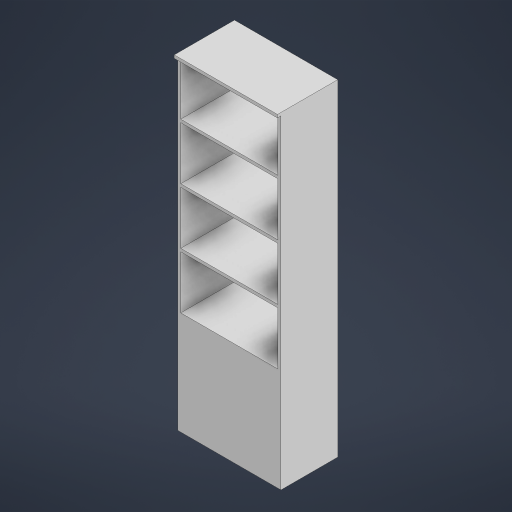
# Autodesk Inventor part: Libreria
Saved by Autodesk Inventor 2024.2 (Build 282272000, 272)
## iProperties
Created: 2025-08-11
Part Number: Libreria
Material: Generic
Document SubType Name: Modeling
Designer: Luca
Density: 1 g/cm^3
Appearance: Default
Author: Luca
Autodesk Inventor part; units mm, degrees
ref_plane "YZ Plane" through (0, 0, 0) normal (1, 0, 0) x (0, 1, 0)
ref_plane "XZ Plane" through (0, 0, 0) normal (0, 1, 0) x (-1, 0, 0)
ref_plane "XY Plane" through (0, 0, 0) normal (0, 0, 1) x (1, 0, 0)
sketch "Sketch1" plane through (0, 0, 0) normal (0, 0, 1) x (1, 0, 0)
  line L0 (-300, 0) -> (300, 0)
  line L1 (300, 0) -> (300, 1900)
  line L2 (300, 1900) -> (-300, 1900)
  line L3 (-300, 1900) -> (-300, 0)
  point P0 (0, 0)
  point P1 (0, 0)
  dimension "d0" = 600
  dimension "d1" = 1900
  constraints: 8 end point, 2 parallel, 1 coincident, 1 horizontal, 1 midpoint, 1 perpendicular
  measures "d0" distance of L0.start L0.end
  measures "d1" distance of L2.end L0.start
extrude "Extrusion1" add sketch "Sketch1" along normal blind 330
sketch "Sketch2" plane through (-300, 1900, 0) normal (0, 1, 0) x (1, 0, 0)
  line L0 (600, 0) -> (0, 0) construction
  line L1 (0, 0) -> (0, -330) construction
  line L2 (600, -330) -> (0, -330) construction
  line L3 (600, 0) -> (600, -330) construction
  line L4 (0, 0) -> (600, 0)
  line L5 (600, 0) -> (600, -350)
  line L6 (600, -350) -> (0, -350)
  line L7 (0, -350) -> (0, 0)
  point P0 (300, 0)
  dimension "d4" = 350
  constraints: 8 end point, 2 parallel, 1 collinear, 1 horizontal, 1 perpendicular
  measures "d4" distance of L6.end L0.end
extrude "Extrusion2" add sketch "Sketch2" against normal blind 17.5
sketch "Sketch3" plane through (0, 0, 330) normal (0, 0, 1) x (1, 0, 0)
  line L0 (300, 1882.5) -> (-300, 1882.5) projected
  line L1 (-282.5, 1882.5) -> (282.5, 1882.5)
  line L2 (282.5, 1882.5) -> (282.5, 1575)
  line L3 (282.5, 1575) -> (-282.5, 1575)
  line L4 (-282.5, 1575) -> (-282.5, 1882.5)
  line L5 (-282.5, 1557.5) -> (282.5, 1557.5)
  line L6 (282.5, 1557.5) -> (282.5, 1250)
  line L7 (282.5, 1250) -> (-282.5, 1250)
  line L8 (-282.5, 1250) -> (-282.5, 1557.5)
  line L9 (282.5, 1232.5) -> (-282.5, 1232.5)
  line L10 (-282.5, 1232.5) -> (-282.5, 925)
  line L11 (-282.5, 925) -> (282.5, 925)
  line L12 (282.5, 925) -> (282.5, 1232.5)
  line L13 (-282.5, 907.5) -> (282.5, 907.5)
  line L14 (282.5, 907.5) -> (282.5, 600)
  line L15 (282.5, 600) -> (-282.5, 600)
  line L16 (-282.5, 600) -> (-282.5, 907.5)
  line L17 (-300, 0) -> (300, 0) projected
  line L18 (-282.5, 1575) -> (-282.5, 1557.5) construction
  line L19 (-282.5, 1250) -> (-282.5, 1232.5) construction
  line L20 (-282.5, 925) -> (-282.5, 907.5) construction
  point P0 (0, 0)
  point P1 (0, 600)
  point P2 (0, 0)
  dimension "d7" = 600
  dimension "d8" = 17.5
  dimension "d9" = 565
  constraints: 38 end point, 10 equal length, 7 point on line, 5 collinear, 4 horizontal, 4 perpendicular, 2 midpoint, 1 vertical, 1 vertical alignment
  measures "d7" distance between parallel lines of L15 L17
  measures "d8" distance of L3.end L5.start
  measures "d9" distance between parallel lines of L2 L4
extrude "Extrusion3" cut sketch "Sketch3" against normal blind 312.5
body "Solid1"
